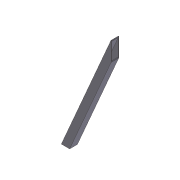
# Autodesk Inventor part: Frame_MainVerticalAngleSupport
Saved by Autodesk Inventor 2012 (Build 160160000, 160)
## iProperties
Created: 2012-01-17
Part Number: Frame_MainVerticalAngleSupport
Material: Aluminum-6061
Document SubType Name: Modeling
Designer: JesseK
Density: 2.71 g/cm^3
Mass: 155.889 g
Surface Area: 730.156 cm^2
Volume: 57.5235 cm^3
Author: JesseK
Autodesk Inventor part; units mm, degrees
ref_plane "YZ Plane" through (0, 0, 0) normal (1, 0, 0) x (0, 1, 0)
ref_plane "XZ Plane" through (0, 0, 0) normal (0, 1, 0) x (-1, 0, 0)
ref_plane "XY Plane" through (0, 0, 0) normal (0, 0, 1) x (1, 0, 0)
sketch "Sketch1" plane through (0, 0, 0) normal (0, 0, 1) x (1, 0, 0)
  line L0 (190.5, 46.6079) -> (218.1822, 46.6079)
  line L1 (218.1822, 46.6079) -> (355.6, 363.7258)
  line L2 (355.6, 363.7258) -> (355.6, 427.6079)
  line L3 (355.6, 427.6079) -> (190.5, 46.6079)
  line L4 (218.1822, 46.6079) -> (355.6, 46.6079) construction
  line L5 (355.6, 46.6079) -> (355.6, 363.7258) construction
  point P0 (0, 0)
  dimension "d0" = 381
  dimension "d2" = 25.4
  dimension "d3" = 165.1
  constraints: 12 end point, 2 horizontal, 2 vertical, 1 parallel
  measures "d0" distance of L4.end L2.end
  measures "d2" distance between parallel lines of L1 L3
  measures "d3" distance of L4.end L0.start
extrude "Extrusion1" add sketch "Sketch1" along normal blind 25.4
shell "Shell1" thickness 1.5875 removed faces 2 at (355.6, 385.0199, 8.4667) at (199.7274, 46.6079, 8.4667)
body "Solid1"
